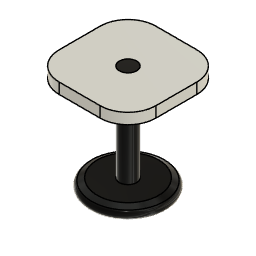
Chair-V1 (Autodesk Fusion 360 design; units mm, degrees)
Autodesk Fusion 360 part; units mm, degrees
sketch "Skizze1" plane through (0, 0, 0) normal (0, 0, 1) x (1, 0, 0)
  circle A0 centre (0, 0) radius 250
  circle A1 centre (0, 0) radius 40
  line L0 (-225, 225) -> (225, 225)
  line L1 (225, 225) -> (225, -225)
  line L2 (225, -225) -> (-225, -225)
  line L3 (-225, -225) -> (-225, 225)
  dimension "d1" = 500
  dimension "d2" = 80
  dimension "d3" = 225
  dimension "d4" = 225
  dimension "d7" = 225
  dimension "d8" = 225
  constraint coincident A0.centre A1.centre
  constraint horizontal L0
  constraint vertical L1
  constraint horizontal L2
  constraint vertical L3
  measures "d1" diameter of A0
  measures "d2" diameter of A1
  measures "d3" distance of A0.centre L3
  measures "d4" distance of A0.centre L1
  measures "d7" distance of A0.centre L0
  measures "d8" distance of A0.centre L2
extrude "Extrusion1" add sketch "Skizze1" along normal blind 50 contours A0 L1 | A0 L0 L1 L2 L3 | A0 L0 | A0 L2 | A0 L3 makes body 1
extrude "Extrusion2" add sketch "Skizze1" along normal blind 500 contours A1 bodies 1
extrude "Extrusion3" add sketch "Skizze1" along normal blind 50 separate body contours A0 L0 L1 L2 L3 | A0 L0 L1 | A0 L1 L2 | A0 L0 L3 | A0 L2 L3 makes body 2
move_body "Verschieben1" bodies 2 to x (1, 0, 0) y (0, 1, 0) z (0, 0, 1) at (0, 0, 800)
move_body "Verschieben2" bodies 2 to x (1, 0, 0) y (0, 1, 0) z (0, 0, 1) at (0, 0, -350)
fillet "Abrundung1" radius 130 4 edges at (225, -225, 475) (-225, -225, 475) (-225, 225, 475) (225, 225, 475) on bodies 2
draft "Verjüngung1" angle -65 neutral plane through (0, 0, 0) pull (0, 0, -1) 1 faces at (-249.6892, 12.4615, 16.6667) on bodies 1
fillet "Abrundung2" radius 20 1 edges at (-233.0818, -90.4039, 0) on bodies 1
